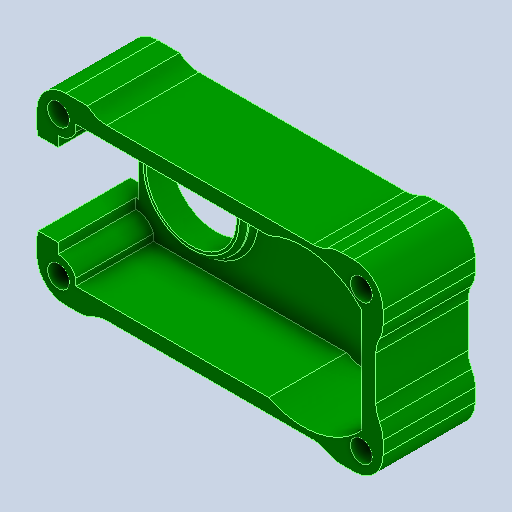
# Autodesk Inventor part: DMS90_Bottom_Plate
Saved by Autodesk Inventor 2023.1 (Build 271208000, 208)
## iProperties
Created: 2022-08-24
Part Number: DMS90_Bottom_Plate
Material: Default New Material
Document SubType Name: Modeling
Designer: Windows10
Density: 1 g/cm^3
Appearance: Generic
Author: Windows10
Autodesk Inventor part; units mm, degrees
ref_plane "YZ Plane" through (0, 0, 0) normal (1, 0, 0) x (0, 1, 0)
ref_plane "XZ Plane" through (0, 0, 0) normal (0, 1, 0) x (-1, 0, 0)
ref_plane "XY Plane" through (0, 0, 0) normal (0, 0, 1) x (1, 0, 0)
sketch "Sketch1" plane through (0, 0, 0) normal (0, 0, 1) x (1, 0, 0)
  line L0 (0, 0) -> (22.85, 0)
  line L1 (22.85, 0) -> (22.85, -11.65)
  line L2 (22.85, -11.65) -> (0, -11.65)
  line L3 (0, -11.65) -> (0, 0)
  dimension "d0" = 22.85
  dimension "d1" = 11.65
  constraints: 8 end point, 2 parallel, 1 horizontal, 1 perpendicular
  measures "d0" distance of L1.end L2.end
  measures "d1" distance of L0.end L1.end
extrude "Extrusion1" add sketch "Sketch1" along normal blind 2
sketch "Sketch2" plane through (0, 0, 2) normal (0, 0, 1) x (1, 0, 0)
  line L0 (0, 0) -> (0, -11.65) projected
  line L1 (0, -5.825) -> (22.85, -5.825)
  line L2 (22.85, -11.65) -> (22.85, 0) projected
  line L3 (0.975, -5.825) -> (21.875, -5.825)
  line L4 (21.875, -5.825) -> (21.875, -0.975)
  line L5 (21.875, -0.975) -> (0.975, -0.975)
  line L6 (0.975, -0.975) -> (0.975, -5.825)
  line L7 (22.85, 0) -> (0, 0) projected
  line L8 (21.875, -5.825) -> (21.875, -10.675)
  line L9 (21.875, -10.675) -> (0.975, -10.675)
  line L10 (0.975, -10.675) -> (0.975, -5.825)
  line L11 (0.975, -1.475) -> (21.875, -1.475)
  line L12 (0.975, -10.175) -> (21.875, -10.175)
  dimension "d4" = 4.85
  dimension "d6" = 0.975
  dimension "d7" = 0.975
  dimension "d8" = 0.5
  constraints: 20 end point, 4 symmetric about line, 3 point on line, 2 midpoint, 2 parallel, 2 perpendicular, 1 horizontal
  measures "d4" distance of L3.end L4.end
  measures "d6" distance between parallel lines of L0 L6
  measures "d7" distance between parallel lines of L2 L4
  measures "d8" distance between parallel lines of L5 L11
extrude "Extrusion2" cut sketch "Sketch2" against normal blind 1 contours L6 L11 L4 L1 | L1 L8 L12 L10
extrude "Extrusion3" [suppressed]
sketch "Sketch3" plane through (0, 0, 2) normal (0, 0, 1) x (1, 0, 0)
  circle A0 centre (1, -1) radius 0.75
  line L0 (22.85, 0) -> (0, 0) projected
  line L1 (0, 0) -> (0, -11.65) projected
  line L2 (11.425, 0) -> (11.425, 1.4162)
  circle A1 centre (21.85, -1) radius 0.75
  line L3 (0, -5.825) -> (-1.2147, -5.825)
  circle A2 centre (1, -10.65) radius 0.75
  circle A3 centre (21.85, -10.65) radius 0.75
  dimension "d13" = 1.5
  dimension "d14" = 1
  dimension "d15" = 1
  constraints: 4 centre point, 4 end point, 3 symmetric about line, 2 midpoint, 1 horizontal, 1 vertical, 3 other
  measures "d13" diameter of A0
  measures "d14" distance from line of L0 A0.centre
  measures "d15" distance from line of L1 A0.centre
extrude "Extrusion4" cut sketch "Sketch3" along normal mid plane 8.25
sketch "Sketch4" plane through (0, 0, 0) normal (0, 0, -1) x (-1, 0, 0)
  circle A0 centre (-1, -10.65) radius 0.75 projected
  circle A1 centre (-21.85, -10.65) radius 0.75 projected
  circle A2 centre (-21.85, -1) radius 0.75 projected
  circle A3 centre (-1, -10.65) radius 0.75 projected
  circle A4 centre (-1, -1) radius 0.75 projected
  line L0 (0, -11.65) -> (-22.85, -11.65) projected
  line L1 (0, 0) -> (0, -11.65) projected
  line L2 (-22.85, 0) -> (0, 0) projected
  line L3 (-22.85, -11.65) -> (-22.85, 0) projected
  circle A5 centre (-1, -10.65) radius 1.5
  line L4 (0, -11.65) -> (-22.85, -11.65) projected
  line L5 (-11.425, -11.65) -> (-11.425, -13.3134)
  line L6 (-22.85, -11.65) -> (-22.85, 0) projected
  line L7 (-22.85, -5.825) -> (-23.9866, -5.825)
  circle A6 centre (-21.85, -10.65) radius 1.5
  circle A7 centre (-1, -1) radius 1.5
  circle A8 centre (-21.85, -1) radius 1.5
  dimension "d18" = 3
  dimension "d21" = 1.5
  constraints: 4 centre point, 4 end point, 3 symmetric about line, 2 midpoint, 1 coincident, 1 horizontal, 1 vertical, 3 other
  measures "d18" diameter of A5
  measures "d21" diameter of A0
extrude "Extrusion5" cut sketch "Sketch4" against normal blind 0.4 contours A0 | A1 | A2 | A4 | L1 A5 L0 | L0 A5 L1 | A7 L2 L1 | L1 L2 A7 | A6 L3 L0 | L0 L3 A6 | A8 L3 L2 | L2 L3 A8
sketch "Sketch5" plane through (0, 0, 0) normal (0, 0, -1) x (-1, 0, 0)
  line L0 (0, -2.118) -> (0, -9.532) projected
  line L1 (0, -5.825) -> (-5.5, -5.825)
  circle A0 centre (-5.5, -5.825) radius 3.1
  point P0 (0, 0)
  dimension "d22" = 5.5
  dimension "d23" = 6.2
  constraints: 2 end point, 1 centre point, 1 coincident, 1 horizontal, 1 midpoint
  measures "d22" distance of L1.start L1.end
  measures "d23" diameter of A0
extrude "Extrusion6" cut sketch "Sketch5" against normal blind 10
sketch "Sketch6" plane through (0, 0, 2) normal (0, 0, 1) x (1, 0, 0)
  arc A0 (1.5804, -1.475) -> (0.975, -1.7496) centre (1, -1) ccw projected
  circle A1 centre (1, -1) radius 1.2915
  arc A2 (21.2696, -10.175) -> (21.875, -9.9004) centre (21.85, -10.65) ccw projected
  line L0 (21.2696, -10.175) -> (1.5804, -10.175) projected
  arc A3 (0.975, -9.9004) -> (1.5804, -10.175) centre (1, -10.65) ccw projected
  line L1 (0.975, -9.9004) -> (0.975, -1.7496) projected
  arc A4 (1.5804, -1.475) -> (0.975, -1.7496) centre (1, -1) ccw projected
  line L2 (1.5804, -1.475) -> (21.2696, -1.475) projected
  arc A5 (21.875, -1.7496) -> (21.2696, -1.475) centre (21.85, -1) ccw projected
  line L3 (21.875, -1.7496) -> (21.875, -9.9004) projected
  line L4 (0, -11.65) -> (22.85, -11.65) projected
  line L5 (22.85, -11.65) -> (22.85, 0) projected
  line L6 (22.85, 0) -> (0, 0) projected
  line L7 (0, 0) -> (0, -11.65) projected
  line L8 (20.732, 0) -> (2.118, 0) projected
  line L9 (11.425, 0) -> (11.425, 0.9871)
  arc A6 (0.975, -1.7496) -> (1.5804, -1.475) centre (1, -1) ccw projected
  line L10 (22.85, -5.825) -> (23.6678, -5.825)
  circle A7 centre (21.85, -1) radius 1.2915
  circle A8 centre (1, -10.65) radius 1.2915
  circle A9 centre (21.85, -10.65) radius 1.2915
  arc A10 (1.5804, -10.175) -> (0.975, -9.9004) centre (1, -10.65) ccw projected
  arc A11 (21.2696, -1.475) -> (21.875, -1.7496) centre (21.85, -1) ccw projected
  arc A12 (21.875, -9.9004) -> (21.2696, -10.175) centre (21.85, -10.65) ccw projected
  point P0 (0.975, -2.2912)
  point P1 (2.201, -1.475)
  point P2 (2.201, -10.175)
  point P3 (0.975, -9.3588)
  point P4 (21.875, -9.3588)
  point P5 (20.649, -10.175)
  point P6 (20.649, -1.475)
  point P7 (21.875, -2.2912)
  constraints: 4 centre point, 4 end point, 3 symmetric about line, 2 midpoint, 1 coincident, 1 horizontal, 1 vertical, 3 other
extrude "Extrusion7" add sketch "Sketch6" against normal blind 1.15 contours L2 A1 L1 A6 | L2 A11 L3 A7 | A8 L0 A10 L1 | L3 A12 L0 A9
sketch "Sketch8" plane through (0, 0, 2) normal (0, 0, 1) x (1, 0, 0)
  line L0 (22.85, 0) -> (0, 0) projected
  line L1 (0, 0) -> (2.5, 0)
  line L2 (2.5, 0) -> (2.5, -2.5)
  line L3 (2.5, -2.5) -> (0, -2.5)
  line L4 (0, -2.5) -> (0, 0)
  line L5 (-0.5, 0.5) -> (3, 0.5)
  line L6 (3, 0.5) -> (3, -3)
  line L7 (3, -3) -> (-0.5, -3)
  line L8 (-0.5, -3) -> (-0.5, 0.5)
  line L9 (0.975, -9.3588) -> (0.975, -2.2912) projected
  arc A0 (0.975, -2.2912) -> (2.201, -1.475) centre (1, -1) ccw projected
  line L10 (2.201, -1.475) -> (20.649, -1.475) projected
  arc A1 (20.649, -1.475) -> (21.875, -2.2912) centre (21.85, -1) ccw projected
  line L11 (21.875, -2.2912) -> (21.875, -9.3588) projected
  arc A2 (21.875, -9.3588) -> (20.649, -10.175) centre (21.85, -10.65) ccw projected
  line L12 (20.649, -10.175) -> (2.201, -10.175) projected
  arc A3 (2.201, -10.175) -> (0.975, -9.3588) centre (1, -10.65) ccw projected
  circle A4 centre (21.85, -10.65) radius 0.75 projected
  circle A5 centre (1, -1) radius 0.75 projected
  circle A6 centre (21.85, -1) radius 0.75 projected
  circle A7 centre (1, -10.65) radius 0.75 projected
  line L13 (0, -11.65) -> (22.85, -11.65) projected
  line L14 (22.85, -11.65) -> (22.85, 0) projected
  line L15 (22.85, 0) -> (0, 0) projected
  line L16 (0, 0) -> (0, -11.65) projected
  line L17 (20.732, 0) -> (2.118, 0) projected
  line L18 (11.425, 0) -> (11.425, 1.8092)
  line L19 (22.85, -9.532) -> (22.85, -2.118) projected
  line L20 (22.85, -5.825) -> (25.3384, -5.825)
  line L21 (22.85, 0) -> (20.35, 0)
  line L22 (20.35, 0) -> (20.35, -2.5)
  line L23 (20.35, -2.5) -> (22.85, -2.5)
  line L24 (22.85, -2.5) -> (22.85, 0)
  line L25 (23.35, 0.5) -> (19.85, 0.5)
  line L26 (19.85, 0.5) -> (19.85, -3)
  line L27 (19.85, -3) -> (23.35, -3)
  line L28 (23.35, -3) -> (23.35, 0.5)
  arc A8 (20.649, -1.475) -> (21.875, -2.2912) centre (21.85, -1) ccw
  circle A9 centre (21.85, -1) radius 0.75
  line L29 (22.85, -11.65) -> (0, -11.65)
  line L30 (0, -11.65) -> (2.5, -11.65)
  line L31 (2.5, -11.65) -> (2.5, -9.15)
  line L32 (2.5, -9.15) -> (0, -9.15)
  line L33 (0, -9.15) -> (0, -11.65)
  line L34 (-0.5, -12.15) -> (3, -12.15)
  line L35 (3, -12.15) -> (3, -8.65)
  line L36 (3, -8.65) -> (-0.5, -8.65)
  line L37 (-0.5, -8.65) -> (-0.5, -12.15)
  arc A10 (2.201, -10.175) -> (0.975, -9.3588) centre (1, -10.65) ccw
  line L38 (2.201, -10.175) -> (20.649, -10.175)
  arc A11 (21.875, -9.3588) -> (20.649, -10.175) centre (21.85, -10.65) ccw
  circle A12 centre (1, -10.65) radius 0.75
  circle A13 centre (21.85, -10.65) radius 0.75
  line L39 (22.85, -11.65) -> (0, -11.65)
  line L40 (20.732, -11.65) -> (2.118, -11.65)
  line L41 (11.425, -11.65) -> (11.425, -13.4592)
  line L42 (22.85, -11.65) -> (20.35, -11.65)
  line L43 (20.35, -11.65) -> (20.35, -9.15)
  line L44 (20.35, -9.15) -> (22.85, -9.15)
  line L45 (22.85, -9.15) -> (22.85, -11.65)
  arc A14 (21.875, -9.3588) -> (20.649, -10.175) centre (21.85, -10.65) ccw
  circle A15 centre (21.85, -10.65) radius 0.75
  line L46 (19.85, -8.65) -> (23.35, -8.65)
  line L47 (23.35, -12.15) -> (19.85, -12.15)
  line L48 (23.35, -8.65) -> (23.35, -12.15)
  line L49 (19.85, -12.15) -> (19.85, -8.65)
  point P0 (0, -3)
  point P1 (3, 0)
  point P2 (19.85, 0)
  point P3 (22.85, -3)
  point P4 (22.85, -8.65)
  point P5 (19.85, -11.65)
  point P6 (3, -11.65)
  point P7 (0, -8.65)
  dimension "d32" = 2.5
  dimension "d33" = 2.5
  dimension "d34" = 0.5
  constraints: 78 end point, 41 symmetric about line, 8 centre point, 8 point on circle, 4 parallel, 2 horizontal, 2 midpoint, 2 perpendicular, 1 vertical, 11 other
  measures "d32" distance of L2.end L3.end
  measures "d33" distance of L1.end L2.end
  measures "d34" distance between parallel lines of L4 L8
extrude "Extrusion9" add sketch "Sketch8" against normal up to surface (1.6 mm away) contours L0 L26 L25 L28 L27 L14 | L0 L4 L16 L7 L8 L5 L6 | L46 L48 L47 L49 L13 L14 | L16 L13 L35 L34 L37 L36
fillet "Fillet1" radius 2 19 edges at (22.85, -3, 1.2) (22.85, -8.65, 1.2) (19.85, 0, 1.2) (19.85, -11.65, 1.2) (3, -11.65, 1.2) (0, -8.65, 1.2) (0, -3, 1.2) (3, 0, 1.2) (-0.5, -3, 1.2) (-0.5, -8.65, 1.2) (3, -12.15, 1.2) (19.85, -12.15, 1.2) (23.35, -8.65, 1.2) (23.35, -3, 1.2) (19.85, 0.5, 1.2) (-0.5, 0.5, 1.2) (-0.5, -12.15, 1.2) (23.35, -12.15, 1.2) (23.35, 0.5, 1.2)
sketch "Sketch9" plane through (0, 0, 1) normal (0, 0, 1) x (1, 0, 0)
  circle A0 centre (5.5, -5.825) radius 3.1 projected
  circle A1 centre (5.5, -5.825) radius 3.6
  point P0 (0, 0)
  dimension "d38" = 0.5
  constraints: 1 centre point, 1 coincident
  measures "d38" radial gap between concentric circles of A0 A1
extrude "Extrusion10" add sketch "Sketch9" along normal blind 0.7
fillet "Fillet2" radius 0.3 2 edges at (1.9, -5.825, 1) (1.9, -5.825, 1.7)
sketch "Sketch10" plane through (0, 0, 2) normal (0, 0, 1) x (1, 0, 0)
  line L0 (2.118, -11.65) -> (20.732, -11.65) projected
  line L1 (20.732, 0) -> (2.118, 0) projected
  line L2 (0, -4.3229) -> (0, -7.3271) projected
  line L3 (22.85, -7.3271) -> (22.85, -4.3229) projected
  line L4 (0, 0) -> (22.85, 0)
  line L5 (22.85, 0) -> (22.85, -11.65)
  line L6 (22.85, -11.65) -> (0, -11.65)
  line L7 (0, -11.65) -> (0, 0)
  line L8 (0, -5.825) -> (25, -5.825)
  circle A0 centre (17.8546, -5.825) radius 5.3813
  arc A1 (20.4636, 0.5) -> (19.4954, 0.25) centre (20.4636, -1.5) ccw projected
  arc A2 (18.5271, 0) -> (19.4954, 0.25) centre (18.5271, 2) ccw projected
  line L9 (18.5271, 0) -> (4.3229, 0) projected
  arc A3 (3, 0.5) -> (4.3229, 0) centre (4.3229, 2) ccw projected
  line L10 (3, 0.5) -> (1.5, 0.5) projected
  arc A4 (1.5, 0.5) -> (-0.5, -1.5) centre (1.5, -1.5) ccw projected
  line L11 (-0.5, -1.5) -> (-0.5, -2.3864) projected
  arc A5 (-0.5, -2.3864) -> (-0.25, -3.3546) centre (1.5, -2.3864) ccw projected
  arc A6 (0, -4.3229) -> (-0.25, -3.3546) centre (-2, -4.3229) ccw projected
  line L12 (0, -4.3229) -> (0, -7.3271) projected
  arc A7 (-0.25, -8.2954) -> (0, -7.3271) centre (-2, -7.3271) ccw projected
  arc A8 (-0.25, -8.2954) -> (-0.5, -9.2636) centre (1.5, -9.2636) ccw projected
  line L13 (-0.5, -9.2636) -> (-0.5, -10.15) projected
  arc A9 (-0.5, -10.15) -> (1.5, -12.15) centre (1.5, -10.15) ccw projected
  line L14 (1.5, -12.15) -> (2.3864, -12.15) projected
  arc A10 (2.3864, -12.15) -> (3.3546, -11.9) centre (2.3864, -10.15) ccw projected
  arc A11 (4.3229, -11.65) -> (3.3546, -11.9) centre (4.3229, -13.65) ccw projected
  line L15 (4.3229, -11.65) -> (18.5271, -11.65) projected
  arc A12 (19.4954, -11.9) -> (18.5271, -11.65) centre (18.5271, -13.65) ccw projected
  arc A13 (19.4954, -11.9) -> (20.4636, -12.15) centre (20.4636, -10.15) ccw projected
  line L16 (20.4636, -12.15) -> (21.35, -12.15) projected
  arc A14 (21.35, -12.15) -> (23.35, -10.15) centre (21.35, -10.15) ccw projected
  line L17 (23.35, -10.15) -> (23.35, -9.2636) projected
  arc A15 (23.35, -9.2636) -> (23.1, -8.2954) centre (21.35, -9.2636) ccw projected
  arc A16 (22.85, -7.3271) -> (23.1, -8.2954) centre (24.85, -7.3271) ccw projected
  line L18 (22.85, -7.3271) -> (22.85, -4.3229) projected
  arc A17 (23.1, -3.3546) -> (22.85, -4.3229) centre (24.85, -4.3229) ccw projected
  arc A18 (23.1, -3.3546) -> (23.35, -2.3864) centre (21.35, -2.3864) ccw projected
  line L19 (23.35, -2.3864) -> (23.35, -1.5) projected
  arc A19 (23.35, -1.5) -> (21.35, 0.5) centre (21.35, -1.5) ccw projected
  line L20 (21.35, 0.5) -> (20.4636, 0.5) projected
  circle A20 centre (1, -10.65) radius 0.75 projected
  circle A21 centre (21.85, -1) radius 0.75 projected
  circle A22 centre (1, -1) radius 0.75 projected
  circle A23 centre (21.85, -10.65) radius 0.75 projected
  line L21 (0.975, -9.3588) -> (0.975, -2.2912) projected
  arc A24 (0.975, -2.2912) -> (2.201, -1.475) centre (1, -1) ccw projected
  line L22 (2.201, -1.475) -> (20.649, -1.475) projected
  arc A25 (20.649, -1.475) -> (21.875, -2.2912) centre (21.85, -1) ccw projected
  line L23 (21.875, -2.2912) -> (21.875, -9.3588) projected
  arc A26 (21.875, -9.3588) -> (20.649, -10.175) centre (21.85, -10.65) ccw projected
  line L24 (20.649, -10.175) -> (2.201, -10.175) projected
  arc A27 (2.201, -10.175) -> (0.975, -9.3588) centre (1, -10.65) ccw projected
  line L25 (21.875, -2.2912) -> (21.875, -2.0373)
  line L26 (21.875, -9.3588) -> (21.875, -9.575)
  line L27 (15.4718, -1) -> (-4, -1)
  line L28 (15.4718, -10.65) -> (-4, -10.65)
  line L29 (2.201, -1.475) -> (2.201, -1)
  line L30 (2.201, -10.175) -> (2.201, -10.65)
  point P0 (14.6866, -1.475)
  point P1 (22.85, -3.8241)
  point P2 (18.5271, 0)
  point P3 (22.85, -7.8259)
  point P4 (14.6866, -10.175)
  point P5 (21.875, -2.2481)
  point P6 (21.875, -9.4019)
  constraints: 22 end point, 4 point on line, 2 horizontal, 2 parallel, 2 perpendicular, 2 symmetric about line, 2 vertical, 1 midpoint, 3 other
extrude "Extrusion11" add sketch "Sketch10" along normal blind 4.35 contours L6 A9 L7 L28 A20 A0 L5 A14 L0 | L0 A11 A10 L14 A9 L6 | L0 L6 A14 L16 A13 A12 | A9 L28 L7 | L28 A9 L13 A8 A7 L7 | L7 L2 L8 L21 A27 L30 L28 A20 | L5 A0 A16 A15 L17 A14 | L2 L7 L27 A22 L29 A24 L21 L8 | A0 L26 L23 L8 L3 L5 | L5 A16 A0 | A6 A5 L11 A4 L27 L7 | L27 A4 L7 | L7 A4 L4 L1 A19 L5 A0 L27 A22 | L8 L23 L25 A0 L5 L3 | L5 A0 A17 | A0 L5 A19 L19 A18 A17 | A4 L10 A3 L1 L4 | L4 L1 A2 A1 L20 A19
sketch "Sketch11" plane through (0, 0, 2) normal (0, 0, 1) x (1, 0, 0)
  line L0 (2.201, -1) -> (2.201, -1.475) projected
  line L1 (2.201, -1.475) -> (20.649, -1.475) projected
  arc A0 (20.649, -1.475) -> (21.875, -2.2912) centre (21.85, -1) ccw projected
  line L2 (21.875, -2.2912) -> (21.875, -2.2481) projected
  arc A1 (21.875, -2.2481) -> (15.4718, -1) centre (17.8546, -5.825) ccw projected
  line L3 (15.4718, -1) -> (2.201, -1) projected
  line L4 (2.201, -10.175) -> (2.201, -10.65) projected
  line L5 (2.201, -10.65) -> (15.4718, -10.65) projected
  arc A2 (15.4718, -10.65) -> (21.875, -9.4019) centre (17.8546, -5.825) ccw projected
  line L6 (21.875, -9.4019) -> (21.875, -9.3588) projected
  arc A3 (21.875, -9.3588) -> (20.649, -10.175) centre (21.85, -10.65) ccw projected
  line L7 (20.649, -10.175) -> (2.201, -10.175) projected
  point P0 (0, 0)
extrude "Extrusion12" cut sketch "Sketch11" against normal up to surface (1 mm away)
sketch "Sketch12" plane through (0, 0, 0.4) normal (0, 0, -1) x (-1, 0, 0)
  arc A0 (-3.3546, -11.9) -> (-2.3864, -12.15) centre (-2.3864, -10.15) ccw projected
  line L0 (-1.5, -12.15) -> (-2.3864, -12.15) projected
  arc A1 (-1.5, -12.15) -> (0.5, -10.15) centre (-1.5, -10.15) ccw projected
  line L1 (0.5, -9.2636) -> (0.5, -10.15) projected
  arc A2 (0.5, -9.2636) -> (0.25, -8.2954) centre (-1.5, -9.2636) ccw projected
  arc A3 (0, -7.3271) -> (0.25, -8.2954) centre (2, -7.3271) ccw projected
  line L2 (0, -9.532) -> (0, -7.3271) projected
  arc A4 (0, -9.532) -> (-2.118, -11.65) centre (-1, -10.65) ccw projected
  line L3 (-4.3229, -11.65) -> (-2.118, -11.65) projected
  arc A5 (-3.3546, -11.9) -> (-4.3229, -11.65) centre (-4.3229, -13.65) ccw projected
  circle A6 centre (-1, -10.65) radius 0.75 projected
  arc A7 (0.25, -3.3546) -> (0.5, -2.3864) centre (-1.5, -2.3864) ccw projected
  line L4 (0.5, -1.5) -> (0.5, -2.3864) projected
  arc A8 (0.5, -1.5) -> (-1.5, 0.5) centre (-1.5, -1.5) ccw projected
  line L5 (-3, 0.5) -> (-1.5, 0.5) projected
  arc A9 (-4.3229, 0) -> (-3, 0.5) centre (-4.3229, 2) ccw projected
  line L6 (-2.118, 0) -> (-4.3229, 0) projected
  arc A10 (-2.118, 0) -> (0, -2.118) centre (-1, -1) ccw projected
  line L7 (0, -4.3229) -> (0, -2.118) projected
  arc A11 (0.25, -3.3546) -> (0, -4.3229) centre (2, -4.3229) ccw projected
  circle A12 centre (-1, -1) radius 0.75 projected
  arc A13 (-19.4954, 0.25) -> (-20.4636, 0.5) centre (-20.4636, -1.5) ccw projected
  line L8 (-21.35, 0.5) -> (-20.4636, 0.5) projected
  arc A14 (-21.35, 0.5) -> (-23.35, -1.5) centre (-21.35, -1.5) ccw projected
  line L9 (-23.35, -2.3864) -> (-23.35, -1.5) projected
  arc A15 (-23.35, -2.3864) -> (-23.1, -3.3546) centre (-21.35, -2.3864) ccw projected
  arc A16 (-22.85, -4.3229) -> (-23.1, -3.3546) centre (-24.85, -4.3229) ccw projected
  line L10 (-22.85, -2.118) -> (-22.85, -4.3229) projected
  arc A17 (-22.85, -2.118) -> (-20.732, 0) centre (-21.85, -1) ccw projected
  line L11 (-18.5271, 0) -> (-20.732, 0) projected
  arc A18 (-19.4954, 0.25) -> (-18.5271, 0) centre (-18.5271, 2) ccw projected
  circle A19 centre (-21.85, -1) radius 0.75 projected
  arc A20 (-23.1, -8.2954) -> (-23.35, -9.2636) centre (-21.35, -9.2636) ccw projected
  line L12 (-23.35, -10.15) -> (-23.35, -9.2636) projected
  arc A21 (-23.35, -10.15) -> (-21.35, -12.15) centre (-21.35, -10.15) ccw projected
  line L13 (-20.4636, -12.15) -> (-21.35, -12.15) projected
  arc A22 (-20.4636, -12.15) -> (-19.4954, -11.9) centre (-20.4636, -10.15) ccw projected
  arc A23 (-18.5271, -11.65) -> (-19.4954, -11.9) centre (-18.5271, -13.65) ccw projected
  line L14 (-20.732, -11.65) -> (-18.5271, -11.65) projected
  arc A24 (-20.732, -11.65) -> (-22.85, -9.532) centre (-21.85, -10.65) ccw projected
  line L15 (-22.85, -7.3271) -> (-22.85, -9.532) projected
  arc A25 (-23.1, -8.2954) -> (-22.85, -7.3271) centre (-24.85, -7.3271) ccw projected
  circle A26 centre (-21.85, -10.65) radius 0.75 projected
  point P0 (0, 0)
extrude "Extrusion13" add sketch "Sketch12" along normal up to surface (0.4 mm away)
sketch "Sketch13" plane through (0, 0, 6.35) normal (0, 0, 1) x (1, 0, 0)
  line L0 (-1.6022, -5.825) -> (1.1857, -5.825)
  line L1 (1.1857, -5.825) -> (1.1857, -3)
  line L2 (1.1857, -3) -> (-1.6022, -3)
  line L3 (-1.6022, -3) -> (-1.6022, -5.825)
  line L4 (1.1857, -5.825) -> (1.1857, -8.65)
  line L5 (1.1857, -8.65) -> (-1.6022, -8.65)
  line L6 (-1.6022, -8.65) -> (-1.6022, -5.825)
  point P0 (0, 0)
  constraints: 14 end point, 2 parallel, 2 symmetric about line, 1 horizontal, 1 perpendicular
extrude "Extrusion14" cut sketch "Sketch13" against normal blind 10
body "Solid1"
